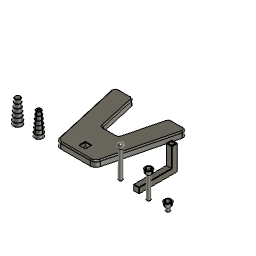
Stativ v5 (Autodesk Fusion 360 design; units mm, degrees)
Autodesk Fusion 360 part; units mm, degrees
sketch "Sketch1" plane through (0, 0, 0) normal (0, 0, 1) x (1, 0, 0) in component "Base"
  line L0 (0, 0) -> (100, 0)
  line L1 (100, 0) -> (148.3195, 194.0753)
  line L2 (148.3195, 194.0753) -> (98.3195, 194.0753)
  line L3 (6.143, 195.1322) -> (-43.857, 195.1322)
  line L4 (-43.857, 195.1322) -> (0, 0)
  line L5 (50, 0) -> (50, 70) construction
  line L6 (29.9173, 89.3536) -> (72.2466, 89.3536)
  line L7 (29.9173, 89.3536) -> (6.143, 195.1322)
  line L8 (98.3195, 194.0753) -> (72.2466, 89.3536)
  dimension "d1" = 50
  dimension "d2" = 50
  dimension "d3" = 100
  dimension "d4" = 200
  dimension "d5" = 200
  dimension "d8" = 70
  dimension "d9" = 91.5826
  dimension "d10" = 108.4174
  dimension "d11" = 107.9186
  dimension "d12" = 42.3293
  dimension "d13" = 103.981
  constraint coincident L0.start L4.end
  constraint horizontal L0
  constraint parallel L0 L2
  constraint parallel L2 L3
  constraint midpoint L0 L5.start
  constraint perpendicular L0 L5
  constraint parallel L0 L6
  measures "d1" distance of L1.end L2.end
  measures "d2" distance of L3.start L3.end
  measures "d3" distance of L0.start L0.end
  measures "d4" distance of L0.end L1.end
  measures "d5" distance of L0.start L3.end
  measures "d8" distance of L5.start L5.end
  measures "d9" distance of L5.start L6.start
  measures "d10" distance of L3.start L6.start
  measures "d11" distance of L2.end L6.end
  measures "d12" distance of L6.start L6.end
  measures "d13" angle of L6 L8
extrude "Extrude1" add sketch "Sketch1" along normal blind 15 makes body 1 in component "Base"
fillet "Fillet1" radius 10 4 edges at (148.3195, 194.0753, 7.5) (6.143, 195.1322, 7.5) (-43.857, 195.1322, 7.5) (98.3195, 194.0753, 7.5) on bodies 1 in component "Base"
fillet "Fillet2" radius 15 2 edges at (0, 0, 7.5) (100, 0, 7.5) on bodies 1 in component "Base"
fillet "Fillet3" radius 5 2 edges at (72.2466, 89.3536, 7.5) (29.9173, 89.3536, 7.5) on bodies 1 in component "Base"
fillet "Fillet4" radius 3 16 edges at (97.5136, 3.1814, 15) (124.0303, 96.5177, 15) (143.4035, 190.2333, 15) (120.8297, 194.0753, 15) (99.9771, 191.9544, 15) (84.811, 139.8184, 15) (71.4178, 90.4141, 15) (51.1286, 89.3536, 15) (30.7943, 90.4496, 15) (18.4688, 140.2911, 15) (4.389, 192.9401, 15) (-16.6094, 195.1322, 15) (-39.1679, 191.38, 15) (-21.8743, 97.325, 15) (2.6311, 3.2881, 15) (50.1398, 0, 15) on bodies 1 in component "Base"
sketch "Sketch1 (1)" plane through (0, 0, 15) normal (0, 0, 1) x (-1, 0, 0) in component "Base"
  arc A0 (-88.2767, -3) -> (-99.9212, -12.1008) centre (-88.2767, -15) ccw
  line L0 (-99.9212, -12.1008) -> (-142.3171, -182.3841)
  arc A1 (-142.3171, -182.3841) -> (-135.5245, -191.0753) centre (-135.5245, -184.0753) ccw
  line L1 (-135.5245, -191.0753) -> (-106.135, -191.0753)
  arc A2 (-106.135, -191.0753) -> (-99.3424, -185.7665) centre (-106.135, -184.0753) ccw
  line L2 (-99.3424, -185.7665) -> (-76.1018, -92.4208)
  arc A3 (-68.3388, -86.3536) -> (-76.1018, -92.4208) centre (-68.3388, -94.3536) ccw
  line L3 (-68.3388, -86.3536) -> (-33.9183, -86.3536)
  arc A4 (-26.113, -92.5993) -> (-33.9183, -86.3536) centre (-33.9183, -94.3536) ccw
  line L4 (-26.113, -92.5993) -> (-4.9707, -186.6672)
  arc A5 (-4.9707, -186.6672) -> (1.8589, -192.1322) centre (1.8589, -185.1322) ccw
  line L5 (1.8589, -192.1322) -> (31.36, -192.1322)
  arc A6 (31.36, -192.1322) -> (38.1896, -183.5972) centre (31.36, -185.1322) ccw
  line L6 (38.1896, -183.5972) -> (-0.2949, -12.3686)
  arc A7 (-0.2949, -12.3686) -> (-12.0029, -3) centre (-12.0029, -15) ccw
  line L7 (-12.0029, -3) -> (-88.2767, -3)
  line L8 (-57.6767, -18) -> (-42.6767, -18)
  line L9 (-42.6767, -18) -> (-42.6767, -33)
  line L10 (-42.6767, -33) -> (-57.6767, -33)
  line L11 (-57.6767, -33) -> (-57.6767, -18)
  line L12 (-88.2767, -3) -> (-88.2767, -73.5732) construction
  line L13 (-12.0029, -3) -> (-12.0029, -72.2348) construction
  dimension "d24" = 15
  dimension "d25" = 15
  dimension "d26" = 15
  dimension "d27" = 30.6
  dimension "d28" = 30.6738
  constraint horizontal L8
  constraint vertical L9
  constraint horizontal L10
  constraint vertical L11
  constraint coincident A0.start L7.end
  constraint perpendicular L7 L12
  constraint coincident A7.end L7.start
  constraint perpendicular L7 L13
  measures "d24" distance of L8.start L8.end
  measures "d25" distance of L8.start L10.end
  measures "d26" distance of L7 L8
  measures "d27" distance of L11 L12
  measures "d28" distance of L9 L13
extrude "Extrude2" cut sketch "Sketch1 (1)" against normal blind 10 contours L8 L9 L10 L11 bodies 1 in component "Base"
sketch "Sketch4" plane through (0, 0, 0) normal (0, 0, 1) x (1, 0, 0) in component "Ring holder"
  circle A0 centre (-100, 0) radius 11.1465
  dimension "d32" = 22.293
  measures "d32" diameter of A0
extrude "Extrude1'" add sketch "Sketch4" along normal blind 10 separate body makes body 2 in component "Ring holder"
sketch "Sketch5" plane through (0, 0, 10) normal (0, 0, 1) x (-1, 0, 0) in component "Ring holder"
  circle A0 centre (100, 0) radius 11.1465
  circle A1 centre (100, 0) radius 10.3503
  dimension "d35" = 20.7006
  constraint concentric A0 A1
  measures "d35" diameter of A1
extrude "Extrude2'" add sketch "Sketch5" along normal blind 10 contours A1 bodies 2 in component "Ring holder"
sketch "Sketch6" plane through (0, 0, 20) normal (0, 0, 1) x (-1, 0, 0) in component "Ring holder"
  circle A0 centre (100, 0) radius 10.3503
  circle A1 centre (100, 0) radius 9.5541
  dimension "d38" = 19.1083
  constraint concentric A0 A1
  measures "d38" diameter of A1
extrude "Extrude3" add sketch "Sketch6" along normal blind 10 contours A1 bodies 2 in component "Ring holder"
sketch "Sketch7" plane through (0, 0, 30) normal (0, 0, 1) x (-1, 0, 0) in component "Ring holder"
  circle A0 centre (100, 0) radius 9.5541
  circle A1 centre (100, 0) radius 8.758
  dimension "d41" = 17.5159
  constraint concentric A0 A1
  measures "d41" diameter of A1
extrude "Extrude4" add sketch "Sketch7" along normal blind 10 contours A1 bodies 2 in component "Ring holder"
sketch "Sketch8" plane through (0, 0, 40) normal (0, 0, 1) x (-1, 0, 0) in component "Ring holder"
  circle A0 centre (100, 0) radius 8.758
  circle A1 centre (100, 0) radius 7.9618
  dimension "d44" = 15.9236
  constraint concentric A0 A1
  measures "d44" diameter of A1
extrude "Extrude5" add sketch "Sketch8" along normal blind 10 contours A1 bodies 2 in component "Ring holder"
sketch "Sketch9" plane through (0, 0, 50) normal (0, 0, 1) x (-1, 0, 0) in component "Ring holder"
  circle A0 centre (100, 0) radius 7.9618
  circle A1 centre (100, 0) radius 7.1656
  dimension "d47" = 14.3312
  constraint concentric A0 A1
  measures "d47" diameter of A1
extrude "Extrude6" add sketch "Sketch9" along normal blind 10 contours A1 bodies 2 in component "Ring holder"
sketch "Sketch1 (2)" plane through (0, 0, 0) normal (0, 0, 1) x (1, 0, 0) in component "Stand"
  line L0 (309.9, 0) -> (325, 0)
  line L1 (325, 0) -> (325, 200)
  line L2 (325, 200) -> (309.9, 200)
  line L3 (309.9, 200) -> (309.9, 0)
  dimension "d50" = 15.1
  dimension "d51" = 200
  constraint horizontal L0
  constraint vertical L1
  constraint horizontal L2
  constraint vertical L3
  measures "d50" distance of L1.end L2.end
  measures "d51" distance of L0.end L1.end
sketch "Sketch2" plane through (0, 0, 15.1) normal (0, 0, 1) x (-1, 0, 0) in component "Stand"
  line L0 (-309.9, -200) -> (-309.9, 0)
  line L1 (-309.9, 0) -> (-325, 0)
  line L2 (-325, 0) -> (-325, -200)
  line L3 (-325, -200) -> (-309.9, -200)
  circle A0 centre (-317.5, -175) radius 5
  dimension "d54" = 10
  dimension "d55" = 25
  dimension "d56" = 7.5
  measures "d54" diameter of A0
  measures "d55" distance of L3 A0.centre
  measures "d56" distance of L2 A0.centre
sketch "Sketch3" plane through (0, 0, 0) normal (0, 0, 1) x (1, 0, 0) in component "Stand"
  line L0 (200, 0) -> (215, 0)
  line L1 (215, 0) -> (215, 100)
  line L2 (215, 100) -> (200, 100)
  line L3 (200, 100) -> (200, 0)
  dimension "d59" = 15
  dimension "d60" = 100
  constraint horizontal L0
  constraint vertical L1
  constraint horizontal L2
  constraint vertical L3
  measures "d59" distance of L0.start L0.end
  measures "d60" distance of L0.start L2.end
extrude "Extrude3'" add sketch "Sketch3" along normal blind 15 separate body makes body 3 in component "Stand"
sketch "Sketch4 (2)" plane through (0, 0, 15) normal (0, 0, 1) x (-1, 0, 0) in component "Stand"
  line L0 (-200, -100) -> (-200, 0)
  line L1 (-200, 0) -> (-215, 0)
  line L2 (-215, 0) -> (-215, -100)
  line L3 (-215, -100) -> (-200, -100)
  line L4 (-200, -100) -> (-215, -100)
  line L5 (-215, -100) -> (-215, -85)
  line L6 (-215, -85) -> (-200, -85)
  line L7 (-200, -85) -> (-200, -100)
  dimension "d63" = 15
  dimension "d64" = 15
  constraint horizontal L4
  constraint vertical L5
  constraint horizontal L6
  constraint vertical L7
  constraint coincident L0.start L3.end
  measures "d63" distance of L0.start L2.end
  measures "d64" distance of L0.start L6.end
extrude "Extrude4'" add sketch "Sketch4 (2)" along normal blind 50 contours L0 L2 L3 L4 L5 L6 L7 bodies 3 in component "Stand"
sketch "Sketch5 (2)" plane through (0, 0, 65) normal (0, 0, 1) x (-1, 0, 0) in component "Stand"
  line L0 (-200, -85) -> (-215, -85)
  line L1 (-215, -85) -> (-215, -100)
  line L2 (-215, -100) -> (-200, -100)
  line L3 (-200, -100) -> (-200, -85)
  circle A0 centre (-207.5, -92.5) radius 5
  dimension "d67" = 10
  measures "d67" diameter of A0
extrude "Extrude5'" cut sketch "Sketch5 (2)" against normal blind 40 contours A0 bodies 3 in component "Stand"
sketch "Sketch1 (3)" plane through (0, 0, 0) normal (0, 1, 0) x (1, 0, 0) in component "Ball"
  line L0 (174.7422, -42.5) -> (179.6922, -42.5)
  line L1 (179.6922, -42.5) -> (179.6922, -114.0626)
  line L2 (174.9765, -112.5) -> (174.7422, -42.5)
  line L3 (175.0013, -119.9146) -> (175.0652, -139) construction
  arc A0 (175.0264, -127.4146) -> (179.6922, -114.0626) centre (175.0013, -119.9146) ccw
  line L4 (175.0013, -119.9146) -> (174.9765, -112.5) construction
  line L5 (175.0264, -127.4146) -> (174.9765, -112.5)
  dimension "d70" = 4.95
  dimension "d73" = 15
  dimension "d109" = 70
  constraint horizontal L0
  constraint perpendicular L0 L1
  constraint coincident L3.start A0.centre
  constraint parallel L2 L4
  constraint coincident L3 A0.start
  constraint parallel L2 L5
  measures "d70" distance of L0.start L0.end
  measures "d73" diameter of A0
  measures "d109" vertical distance of L0.start L2.start
revolve "Revolve1" add sketch "Sketch1 (3)" angle 360 about axis through (174.9765, 0, 112.5) along (-0.003347, 0, -0.999994) separate body makes body 4 in component "Ball"
sketch "Sketch10" plane through (0, 0, 0) normal (0, 0, -1) x (1, 0, 0) in component "Ring holder"
  circle A0 centre (-100, 0) radius 11.1465
  circle A1 centre (-100, 0) radius 5
  dimension "d75" = 10
  constraint concentric A0 A1
  measures "d75" diameter of A1
extrude "Extrude7" cut sketch "Sketch10" against normal blind 50 contours A1 bodies 2 in component "Ring holder"
sketch "Sketch1 (4)" plane through (0, 0, 0) normal (0, 1, 0) x (1, 0, 0) in component "Joint"
  line L0 (240, 0) -> (240, -59.428)
  line L1 (240, 0) -> (244.95, 0)
  line L2 (244.95, -58.2391) -> (244.95, 0)
  arc A0 (249.5394, -69.928) -> (244.95, -58.2391) centre (240, -66.928) ccw
  arc A1 (246.8739, -69.928) -> (240, -59.428) centre (240, -66.928) ccw
  line L3 (246.8739, -69.928) -> (249.5394, -69.928) construction
  line L4 (246.8739, -69.928) -> (249.5394, -69.928)
  dimension "d80" = 4.95
  dimension "d81" = 20
  dimension "d82" = 15
  constraint vertical L0
  constraint perpendicular L0 L1
  constraint concentric A0 A1
  measures "d80" distance of L0.start L1.end
  measures "d81" diameter of A0
  measures "d82" diameter of A1
revolve "Revolve1'" add sketch "Sketch1 (4)" angle 360 about axis through (240, 0, 0) along (0, 0, 1) separate body makes body 5 in component "Joint"
sketch "Sketch2 (2)" plane through (0, 0, 69.928) normal (0, 0, 1) x (-1, 0, 0) in component "Joint"
  circle A0 centre (-240, 0) radius 9.5394
  circle A1 centre (-240, 0) radius 6.8739
  line L0 (-230.4606, 0.0002) -> (-249.5394, 0.0002) construction
  line L1 (-240, 0) -> (-240, 9.7088) construction
  line L2 (-240, 9.7088) -> (-240, -9.5394) construction
  line L3 (-238.5, -12.5) -> (-241.5, -12.5)
  line L4 (-241.5, -12.5) -> (-241.5, 12.5)
  line L5 (-241.5, 12.5) -> (-238.5, 12.5)
  line L6 (-238.5, 12.5) -> (-238.5, -12.5)
  line L7 (-227.5, -1.4998) -> (-252.5, -1.4998)
  line L8 (-252.5, -1.4998) -> (-252.5, 1.5002)
  line L9 (-252.5, 1.5002) -> (-227.5, 1.5002)
  line L10 (-227.5, 1.5002) -> (-227.5, -1.4998)
  dimension "d85" = 3
  dimension "d86" = 25
  dimension "d87" = 25
  dimension "d88" = 3
  dimension "d89" = 1.5
  dimension "d90" = 1.5
  dimension "d91" = 12.5
  dimension "d92" = 12.5
  constraint coincident A0 L0.start
  constraint coincident A0 L0.end
  constraint horizontal L0
  constraint coincident A0.centre A1.centre
  constraint perpendicular L0 L1
  constraint coincident A0 L2.end
  constraint perpendicular L0 L2
  constraint horizontal L3
  constraint vertical L4
  constraint horizontal L5
  constraint vertical L6
  constraint horizontal L7
  constraint vertical L8
  constraint horizontal L9
  constraint vertical L10
  measures "d85" distance of L3.start L3.end
  measures "d86" distance of L3.start L5.end
  measures "d87" distance of L7.start L7.end
  measures "d88" distance of L7.start L9.end
  measures "d89" distance of L0 L7
  measures "d90" distance of L2 L4
  measures "d91" distance of A0.centre L10
  measures "d92" distance of A0.centre L3
extrude "Extrude1''" cut sketch "Sketch2 (2)" against normal blind 8 contours A0 A1 L7 L9 | A0 L7 L9 L10 | A0 A1 L4 L6 | A0 L4 L5 L6 | A1 L6 L7 L9 | A0 L3 L4 L6 | A0 A1 L4 L6 | A1 L4 L6 L9 | L4 L6 L7 L9 | A1 L4 L6 L7 | A0 A1 L7 L9 | A0 L7 L8 L9 | A1 L4 L7 L9 bodies 5 in component "Joint"
fillet "Fillet1'" radius 1 8 edges at (215, 42.5, 15) (215, 50, 0) (200, 42.5, 15) (200, 50, 0) (200, 0, 7.5) (207.5, 0, 15) (215, 0, 7.5) (207.5, 0, 0) on bodies 3 in component "Stand"
fillet "Fillet1'" radius 1 9 edges at (200, 100, 32.5) (200, 85, 40) (215, 85, 40) (215, 100, 32.5) (215, 92.5, 65) (207.5, 100, 65) (200, 92.5, 65) (207.5, 85, 65) (212.1616, 90.6919, 65) on bodies 3 in component "Stand"
fillet "Fillet1''" radius 1 1 edges at (235.385, -1.79, 0) on bodies 5 in component "Joint"
fillet "Fillet1'''" radius 1 1 edges at (170.1273, -1.79, 42.532) on bodies 4 in component "Ball"
fillet "Fillet1''''" radius 1 3 edges at (-110.3922, -4.0307, 0) (-93.3193, 2.5912, 60) (-104.6616, -1.8081, 0) on bodies 2 in component "Ring holder"
fillet "Fillet1''''" radius 0.3 5 edges at (-92.577, 2.8791, 50) (-91.8347, 3.167, 40) (-91.0924, 3.4549, 30) (-90.3501, 3.7428, 20) (-110.3922, -4.0307, 10) on bodies 2 in component "Ring holder"
fillet "Fillet5" radius 1 4 edges at (50.1767, 33, 15) (57.6767, 25.5, 15) (42.6767, 25.5, 15) (50.1767, 18, 15) on bodies 1 in component "Base"
sketch "Sketch4 (3)" plane through (0, 0, 0) normal (0, 0, 1) x (1, 0, 0) in component "Mandrel"
  circle A0 centre (-100, 0) radius 10.6465
  dimension "d32_1" = 21.293
  measures "d32_1" diameter of A0
extrude "Extrude1'''" add sketch "Sketch4 (3)" along normal blind 10 separate body makes body 6 in component "Mandrel"
sketch "Sketch5 (3)" plane through (0, 0, 10) normal (0, 0, 1) x (-1, 0, 0) in component "Mandrel"
  circle A0 centre (100, 0) radius 10.6465
  circle A1 centre (100, 0) radius 9.8503
  dimension "d35_1" = 19.7006
  constraint concentric A0 A1
  measures "d35_1" diameter of A1
extrude "Extrude2''" add sketch "Sketch5 (3)" along normal blind 10 contours A1 bodies 6 in component "Mandrel"
sketch "Sketch6 (2)" plane through (0, 0, 20) normal (0, 0, 1) x (-1, 0, 0) in component "Mandrel"
  circle A0 centre (100, 0) radius 9.8503
  circle A1 centre (100, 0) radius 9.0541
  dimension "d38_1" = 18.1083
  constraint concentric A0 A1
  measures "d38_1" diameter of A1
extrude "Extrude3''" add sketch "Sketch6 (2)" along normal blind 10 contours A1 bodies 6 in component "Mandrel"
sketch "Sketch7 (2)" plane through (0, 0, 30) normal (0, 0, 1) x (-1, 0, 0) in component "Mandrel"
  circle A0 centre (100, 0) radius 9.0541
  circle A1 centre (100, 0) radius 8.258
  dimension "d41_1" = 16.5159
  constraint concentric A0 A1
  measures "d41_1" diameter of A1
extrude "Extrude4''" add sketch "Sketch7 (2)" along normal blind 10 contours A1 bodies 6 in component "Mandrel"
sketch "Sketch8 (2)" plane through (0, 0, 40) normal (0, 0, 1) x (-1, 0, 0) in component "Mandrel"
  circle A0 centre (100, 0) radius 8.258
  circle A1 centre (100, 0) radius 7.4618
  dimension "d44_1" = 14.9236
  constraint concentric A0 A1
  measures "d44_1" diameter of A1
extrude "Extrude5''" add sketch "Sketch8 (2)" along normal blind 10 contours A1 bodies 6 in component "Mandrel"
sketch "Sketch9 (2)" plane through (0, 0, 50) normal (0, 0, 1) x (-1, 0, 0) in component "Mandrel"
  circle A0 centre (100, 0) radius 7.4618
  circle A1 centre (100, 0) radius 6.6656
  dimension "d47_1" = 13.3312
  constraint concentric A0 A1
  measures "d47_1" diameter of A1
extrude "Extrude6'" add sketch "Sketch9 (2)" along normal blind 10 contours A1 bodies 6 in component "Mandrel"
sketch "Sketch10 (2)" plane through (0, 0, 0) normal (0, 0, -1) x (1, 0, 0) in component "Mandrel"
  circle A0 centre (-100, 0) radius 10.6465
  circle A1 centre (-100, 0) radius 5
  dimension "d75_1" = 10
  constraint concentric A0 A1
  measures "d75_1" diameter of A1
extrude "Extrude7'" cut sketch "Sketch10 (2)" against normal blind 50 contours A1 bodies 6 in component "Mandrel"
fillet "Fillet1'''''" radius 1 3 edges at (-109.926, -3.8499, 0) (-93.7855, 2.4104, 60) (-104.6616, -1.8081, 0) on bodies 6 in component "Mandrel"
fillet "Fillet1'''''" radius 0.3 5 edges at (-93.0432, 2.6983, 50) (-92.3009, 2.9862, 40) (-91.5586, 3.2741, 30) (-90.8163, 3.562, 20) (-109.926, -3.8499, 10) on bodies 6 in component "Mandrel"
sketch "Sketch11" plane through (0, 0, 60) normal (0, 0, 1) x (-1, 0, 0) in component "Mandrel"
  circle A0 centre (100, 0) radius 5.6656
  line L0 (115, -0.5) -> (85, -0.5)
  line L1 (85, -0.5) -> (85, 0.5)
  line L2 (85, 0.5) -> (115, 0.5)
  line L3 (115, 0.5) -> (115, -0.5)
  line L4 (100, 0) -> (105.6656, 0) construction
  line L5 (100, 0) -> (100, -5.6656) construction
  line L6 (100.5, -15) -> (99.5, -15)
  line L7 (99.5, -15) -> (99.5, 15)
  line L8 (99.5, 15) -> (100.5, 15)
  line L9 (100.5, 15) -> (100.5, -15)
  dimension "d111" = 30
  dimension "d112" = 1
  dimension "d113" = 0.5
  dimension "d114" = 15
  dimension "d115" = 1
  dimension "d116" = 30
  dimension "d117" = 0.5
  dimension "d118" = 15
  constraint horizontal L0
  constraint vertical L1
  constraint horizontal L2
  constraint vertical L3
  constraint coincident A0.centre L4.start
  constraint coincident A0 L4.end
  constraint horizontal L4
  constraint coincident A0 L5.end
  constraint perpendicular L4 L5
  constraint horizontal L6
  constraint vertical L7
  constraint horizontal L8
  constraint vertical L9
  measures "d111" distance of L0.start L0.end
  measures "d112" distance of L0.start L2.end
  measures "d113" distance of L0 A0.centre
  measures "d114" distance of L3 A0.centre
  measures "d115" distance of L6.start L6.end
  measures "d116" distance of L6.start L8.end
  measures "d117" distance of A0.centre L7
  measures "d118" distance of A0.centre L6
extrude "Extrude8" cut sketch "Sketch11" against normal blind 50 contours A0 L0 L2 L9 | A0 L0 L2 L3 | A0 L2 L7 L9 | A0 L7 L8 L9 | L0 L2 L7 L9 | A0 L6 L7 L9 | A0 L0 L7 L9 | A0 L0 L2 L7 | A0 L0 L1 L2 bodies 6 in component "Mandrel"
sketch "Sketch1 (5)" plane through (0, 0, 0) normal (0, 1, 0) x (1, 0, 0) in component "Joint (1)"
  line L0 (240, 0) -> (240, -11.1889)
  line L1 (240, 0) -> (244.95, 0)
  line L2 (244.95, -10) -> (244.95, 0)
  arc A0 (249.5394, -21.6889) -> (244.95, -10) centre (240, -18.6889) ccw
  arc A1 (246.8739, -21.6889) -> (240, -11.1889) centre (240, -18.6889) ccw
  line L3 (246.8739, -21.6889) -> (249.5394, -21.6889) construction
  line L4 (246.8739, -21.6889) -> (249.5394, -21.6889)
  dimension "d80_1" = 4.95
  dimension "d81_1" = 20
  dimension "d82_1" = 15
  dimension "d121" = 10
  constraint vertical L0
  constraint perpendicular L0 L1
  constraint concentric A0 A1
  measures "d80_1" distance of L0.start L1.end
  measures "d81_1" diameter of A0
  measures "d82_1" diameter of A1
  measures "d121" distance of L1.end L2.start
revolve "Revolve1''" add sketch "Sketch1 (5)" angle 360 about axis through (240, 0, 0) along (0, 0, 1) separate body makes body 7 in component "Joint (1)"
sketch "Sketch2 (3)" plane through (0, 0, 21.6889) normal (0, 0, 1) x (-1, 0, 0) in component "Joint (1)"
  circle A0 centre (-240, 0) radius 9.5394
  circle A1 centre (-240, 0) radius 6.8739
  line L0 (-230.4606, 0.0002) -> (-249.5394, 0.0002) construction
  line L1 (-240, 0) -> (-240, 9.7088) construction
  line L2 (-240, 9.7088) -> (-240, -9.5394) construction
  line L3 (-238.5, -12.5) -> (-241.5, -12.5)
  line L4 (-241.5, -12.5) -> (-241.5, 12.5)
  line L5 (-241.5, 12.5) -> (-238.5, 12.5)
  line L6 (-238.5, 12.5) -> (-238.5, -12.5)
  line L7 (-227.5, -1.4998) -> (-252.5, -1.4998)
  line L8 (-252.5, -1.4998) -> (-252.5, 1.5002)
  line L9 (-252.5, 1.5002) -> (-227.5, 1.5002)
  line L10 (-227.5, 1.5002) -> (-227.5, -1.4998)
  dimension "d85_1" = 3
  dimension "d86_1" = 25
  dimension "d87_1" = 25
  dimension "d88_1" = 3
  dimension "d89_1" = 1.5
  dimension "d90_1" = 1.5
  dimension "d91_1" = 12.5
  dimension "d92_1" = 12.5
  constraint coincident A0 L0.start
  constraint coincident A0 L0.end
  constraint horizontal L0
  constraint coincident A0.centre A1.centre
  constraint perpendicular L0 L1
  constraint coincident A0 L2.end
  constraint perpendicular L0 L2
  constraint horizontal L3
  constraint vertical L4
  constraint horizontal L5
  constraint vertical L6
  constraint horizontal L7
  constraint vertical L8
  constraint horizontal L9
  constraint vertical L10
  measures "d85_1" distance of L3.start L3.end
  measures "d86_1" distance of L3.start L5.end
  measures "d87_1" distance of L7.start L7.end
  measures "d88_1" distance of L7.start L9.end
  measures "d89_1" distance of L0 L7
  measures "d90_1" distance of L2 L4
  measures "d91_1" distance of A0.centre L10
  measures "d92_1" distance of A0.centre L3
extrude "Extrude1''''" cut sketch "Sketch2 (3)" against normal blind 8 contours A0 A1 L7 L9 | A0 L7 L9 L10 | A0 A1 L4 L6 | A0 L4 L5 L6 | A1 L6 L7 L9 | A0 L3 L4 L6 | A0 A1 L4 L6 | A1 L4 L6 L9 | L4 L6 L7 L9 | A1 L4 L6 L7 | A0 A1 L7 L9 | A0 L7 L8 L9 | A1 L4 L7 L9 bodies 7 in component "Joint (1)"
fillet "Fillet1''''''" radius 1 1 edges at (235.385, -1.79, 0) on bodies 7 in component "Joint (1)"
component "Base" placed x (1, 0, 0) y (0, 1, 0) z (0, 0, 1) at (0, 0, 0)
component "Stand" placed x (1, 0, 0) y (0, 1, 0) z (0, 0, 1) at (0, 0, 0)
component "Ring holder" placed x (1, 0, 0) y (0, 1, 0) z (0, 0, 1) at (0, 0, 0)
component "Ball" placed x (1, 0, 0) y (0, 1, 0) z (0, 0, 1) at (-16.3125, 8.3939, -42.5068)
component "Joint" placed x (1, 0, 0) y (0, 1, 0) z (0, 0, 1) at (0, 0, 0)
component "Mandrel" placed x (1, 0, 0) y (0, 1, 0) z (0, 0, 1) at (55, 0, 0)
component "Joint (1)" placed x (1, 0, 0) y (0, 1, 0) z (0, 0, 1) at (0, 0, 0)
equation "d32 = ( 70 / 3.14 ) * 1 mm"
equation "d35 = ( 65 / 3.14 ) * 1 mm"
equation "d38 = ( 60 / 3.14 ) * 1 mm"
equation "d41 = ( 55 / 3.14 ) * 1 mm"
equation "d44 = ( 50 / 3.14 ) * 1 mm"
equation "d47 = ( 45 / 3.14 ) * 1 mm"
equation "d70 = ( 9.9 / 2 ) * 1 mm"
equation "d91 = ( 25 / 2 ) * 1 mm"
equation "d92 = ( 25 / 2 ) * 1 mm"
equation "d32_1 = ( ( 70 / 3.14 ) * 1 mm ) - 1 mm"
equation "d35_1 = ( ( 65 / 3.14 ) * 1 mm ) - 1 mm"
equation "d38_1 = ( ( 60 / 3.14 ) * 1 mm ) - 1 mm"
equation "d41_1 = ( ( 55 / 3.14 ) * 1 mm ) - 1 mm"
equation "d44_1 = ( ( 50 / 3.14 ) * 1 mm ) - 1 mm"
equation "d47_1 = ( ( 45 / 3.14 ) * 1 mm ) - 1 mm"
equation "d91_1 = ( 25 / 2 ) * 1 mm"
equation "d92_1 = ( 25 / 2 ) * 1 mm"
